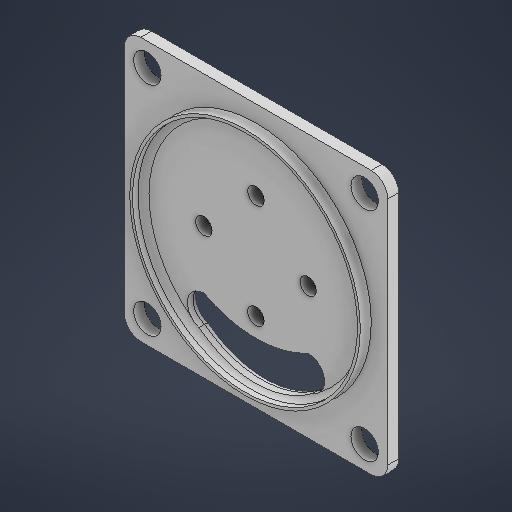
# Autodesk Inventor part: КрашкаКорпДвиг
Saved by Autodesk Inventor 2026 (Build 300175000, 175)
## iProperties
Created: 2025-08-20
Part Number: КрашкаКорпДвиг
Material: Типовые
Document SubType Name: Modeling
Designer: seraf
Density: 1 g/cm^3
Appearance: По умолчанию
Author: seraf
Autodesk Inventor part; units mm, degrees
ref_plane "YZ Plane" through (0, 0, 0) normal (1, 0, 0) x (0, 1, 0)
ref_plane "XZ Plane" through (0, 0, 0) normal (0, 1, 0) x (-1, 0, 0)
ref_plane "XY Plane" through (0, 0, 0) normal (0, 0, 1) x (1, 0, 0)
sketch "Эскиз1" plane through (0, 0, 0) normal (0, 0, 1) x (1, 0, 0)
  line L0 (-24, -24) -> (24, -24)
  line L1 (24, -24) -> (24, 24)
  line L2 (24, 24) -> (-24, 24)
  line L3 (-24, 24) -> (-24, -24)
  line L4 (-24, -24) -> (24, 24) construction
  line L5 (24, -24) -> (-24, 24) construction
  circle A0 centre (-19.799, 19.799) radius 2.5
  line L6 (0, 0) -> (-19.799, 19.799) construction
  circle A1 centre (-19.799, -19.801) radius 2.5
  circle A2 centre (19.801, 19.799) radius 2.5
  circle A3 centre (19.801, -19.801) radius 2.5
  circle A4 centre (0, 0) radius 9.5 construction
  circle A5 centre (9.5, 0) radius 1.5
  circle A6 centre (0, 9.5) radius 1.5
  circle A7 centre (-9.5, 0) radius 1.5
  circle A8 centre (0, -9.5) radius 1.5
  line L7 (0, 24) -> (0, -24)
  line L8 (-24, 0) -> (24, 0)
  line L9 (9.5, -16.5997) -> (9.5, -10.5997) construction
  line L10 (-9.5, -10.5997) -> (-9.5, -16.5997) construction
  line L11 (-9.5, -16.5997) -> (9.5, -10.5997) construction
  line L12 (9.5, -16.5997) -> (-9.5, -10.5997) construction
  arc A9 (-9.5, -10.5997) -> (-10.3701, -16.4708) centre (-9.5, -13.5997) ccw
  arc A10 (10.3701, -16.4708) -> (9.5, -10.5997) centre (9.5, -13.5997) ccw
  arc A11 (-10.3701, -16.4708) -> (10.3701, -16.4708) centre (0, -3) ccw
  arc A12 (-9.5, -10.5997) -> (9.5, -10.5997) centre (0, 7) ccw
  point P0 (0, -13.5997)
  point P1 (0, -17)
  point P2 (0, -12.5)
  point P3 (0, -20)
  dimension "d0" = 48
  dimension "d1" = 48
  dimension "d2" = 5
  dimension "d3" = 28
  dimension "d6" = 39.6
  dimension "d9" = 39.6
  dimension "d12" = 19
  dimension "d13" = 3
  dimension "d14" = 3
  dimension "d15" = 3
  dimension "d17" = 19
  dimension "d18" = 6
  dimension "d24" = 20
  dimension "d25" = 3
  dimension "d26" = 2
  dimension "d35" = 4
  dimension "d37" = 17
  constraints: 26 end point, 13 centre point, 13 point on circle, 10 midpoint, 9 point on line, 3 parallel, 2 horizontal, 2 perpendicular, 1 coincident, 1 vertical, 6 other
  measures "d0" distance of L2.end L1.end
  measures "d1" distance of L1.end L0.end
  measures "d2" diameter of A0
  measures "d3" distance of L6.end L6.start
  measures "d6" distance of L6.end A1.centre
  measures "d9" distance of L6.end A2.centre
  measures "d12" diameter of A4
  measures "d13" diameter of A5
  measures "d14" diameter of A6
  measures "d15" diameter of A7
  measures "d17" distance of L10.start L9.end
  measures "d18" distance of L9.end L9.start
  measures "d24" radius of A12
  measures "d25" diameter of A8
  measures "d35" distance of L7.end point (0, -20)
  measures "d37" radius of A11
extrude "Выдавливание1" add sketch "Эскиз1" along normal blind 2 contours L3 L8 A7 L7 A8 A12 A9 A11 L0 | L7 A11 A10 A12 A8 L8 A5 L1 L0 | L3 L2 L7 A6 L8 A7 | L8 A5 L7 A6 L2 L1
fillet "Сопряжение1" radius 3 4 edges at (-24, -24, 1) (24, -24, 1) (-24, 24, 1) (24, 24, 1)
sketch "Эскиз2" plane through (0, 0, 2) normal (0, 0, 1) x (1, 0, 0)
  circle A0 centre (0, 0) radius 21
  circle A1 centre (0, 0) radius 20.5
  dimension "d30" = 42
  dimension "d31" = 41
  constraints: 2 centre point, 2 coincident
  measures "d30" diameter of A0
  measures "d31" diameter of A1
extrude "Выдавливание2" add sketch "Эскиз2" along normal blind 2
fillet "Сопряжение2" radius 1 1 edges at (-20.5, 0, 2)
fillet "Сопряжение3" radius 1 4 edges at (0, -13, 0) (-12.4676, -13.1599, 0) (0, -20, 0) (12.4676, -13.1599, 0)
